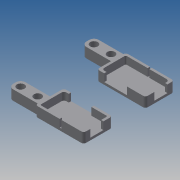
# Autodesk Inventor part: Limit Switch Mount Mount
Saved by Autodesk Inventor 2014 SP1 (Build 180222100, 222)
## iProperties
Created: 2014-02-14
Part Number: Limit Switch Mount Mount
Material: Generic
Document SubType Name: Modeling
Designer: Pradhan Alexander
Density: 1 g/cm^3
Appearance: Default
Author: Pradhan Alexander
Autodesk Inventor part; units mm, degrees
ref_plane "YZ Plane" through (0, 0, 0) normal (1, 0, 0) x (0, 1, 0)
ref_plane "XZ Plane" through (0, 0, 0) normal (0, 1, 0) x (-1, 0, 0)
ref_plane "XY Plane" through (0, 0, 0) normal (0, 0, 1) x (1, 0, 0)
sketch "Sketch1" plane through (0, 0, 0) normal (0, 1, 0) x (-1, 0, 0)
  line L0 (-4.3352, 9.4071) -> (21.4966, 9.4071)
  line L1 (23.2873, 7.6164) -> (23.2873, -4.8804)
  line L2 (20.7346, -6.5949) -> (-4.3352, -6.5949)
  line L3 (-5.9227, -5.0074) -> (-5.9227, 7.8196)
  line L4 (-5.9227, 10.9946) -> (23.2873, 10.9946)
  line L5 (24.8748, 9.4071) -> (24.8748, -6.5949)
  line L6 (23.2873, -8.1824) -> (-5.9227, -8.1824)
  line L7 (-7.5102, -6.5949) -> (-7.5102, 9.4071)
  arc A0 (-5.9227, -5.0074) -> (-4.3352, -6.5949) centre (-4.3352, -5.0074) ccw
  arc A1 (23.2873, 7.6164) -> (21.4966, 9.4071) centre (21.4966, 7.6164) ccw
  arc A2 (-7.5102, -6.5949) -> (-5.9227, -8.1824) centre (-5.9227, -6.5949) ccw
  arc A3 (-5.9227, 10.9946) -> (-7.5102, 9.4071) centre (-5.9227, 9.4071) ccw
  arc A4 (24.8748, 9.4071) -> (23.2873, 10.9946) centre (23.2873, 9.4071) ccw
  arc A5 (23.2873, -8.1824) -> (24.8748, -6.5949) centre (23.2873, -6.5949) ccw
  line L8 (-4.3352, 9.4071) -> (-5.129, 9.4071)
  line L9 (-5.9227, 8.6134) -> (-5.9227, 7.8196)
  line L10 (20.7346, -6.5949) -> (22.4935, -6.5949)
  line L11 (23.2873, -5.8011) -> (23.2873, -4.8804)
  arc A6 (22.4935, -6.5949) -> (23.2873, -5.8011) centre (22.4935, -5.8011) ccw
  arc A7 (-5.129, 9.4071) -> (-5.9227, 8.6134) centre (-5.129, 8.6134) ccw
  point P0 (-5.9227, 9.4071)
  point P1 (-5.9227, -6.5949)
  dimension "d0" = 16.002
  dimension "d2" = 1.5875
  dimension "d3" = 1.5875
  dimension "d4" = 1.5875
  dimension "d5" = 1.5875
  dimension "d31" = 0.7937
  dimension "d45" = 29.21
  constraints: 24 end point, 16 point on circle, 16 tangent, 10 point on line, 8 centre point, 4 parallel, 4 perpendicular, 2 equal radius, 2 horizontal, 1 collinear
  measures "d0" distance of point (-5.923, -6.595) point (-5.923, 9.407)
  measures "d2" distance between parallel lines of L3 L7
  measures "d3" distance between parallel lines of L5 L1
  measures "d4" distance between parallel lines of L6 L2
  measures "d5" distance between parallel lines of L0 L4
  measures "d31" radius of A6
  measures "d45" distance between parallel lines of L1 L3
extrude "Extrusion1" add sketch "Sketch1" along normal blind 6.35 contours L0 A1 L1 L11 A6 L10 L2 A0 L3 L9 A7 L8 | L4 A4 L5 A5 L6 A2 L7 A3
sketch "Sketch3" plane through (0, 6.35, 0) normal (0, 1, 0) x (1, 0, 0)
  line L0 (7.5102, -9.4071) -> (7.5102, 6.5949) projected
  arc A0 (7.5102, 6.5949) -> (5.9227, 8.1824) centre (5.9227, 6.5949) ccw projected
  line L1 (5.9227, 8.1824) -> (-23.2873, 8.1824) projected
  arc A1 (-23.2873, 8.1824) -> (-24.8748, 6.5949) centre (-23.2873, 6.5949) ccw projected
  line L2 (-24.8748, 6.5949) -> (-24.8748, -9.4071) projected
  arc A2 (-24.8748, -9.4071) -> (-23.2873, -10.9946) centre (-23.2873, -9.4071) ccw projected
  line L3 (-23.2873, -10.9946) -> (5.9227, -10.9946) projected
  arc A3 (5.9227, -10.9946) -> (7.5102, -9.4071) centre (5.9227, -9.4071) ccw projected
  line L4 (-4.3352, 6.5949) -> (4.132, 6.5949)
  line L5 (5.9227, 4.8042) -> (5.9227, -7.6926)
  line L6 (4.005, -9.4071) -> (-21.6998, -9.4071)
  line L7 (-23.2873, -7.8196) -> (-23.2873, 5.0074)
  line L8 (-23.2873, 8.1824) -> (5.9227, 8.1824)
  line L9 (7.5102, 6.5949) -> (7.5102, -9.4071)
  line L10 (5.9227, -10.9946) -> (-23.2873, -10.9946)
  line L11 (-24.8748, -9.4071) -> (-24.8748, 6.5949)
  arc A4 (-23.2873, -7.8196) -> (-21.6998, -9.4071) centre (-21.6998, -7.8196) ccw
  arc A5 (5.9227, 4.8042) -> (4.132, 6.5949) centre (4.132, 4.8042) ccw
  arc A6 (-24.8748, -9.4071) -> (-23.2873, -10.9946) centre (-23.2873, -9.4071) ccw
  arc A7 (-23.2873, 8.1824) -> (-24.8748, 6.5949) centre (-23.2873, 6.5949) ccw
  arc A8 (7.5102, 6.5949) -> (5.9227, 8.1824) centre (5.9227, 6.5949) ccw
  arc A9 (5.9227, -10.9946) -> (7.5102, -9.4071) centre (5.9227, -9.4071) ccw
  line L12 (-4.3352, 6.5949) -> (-22.4935, 6.5949)
  line L13 (-23.2873, 5.8011) -> (-23.2873, 5.0074)
  line L14 (4.005, -9.4071) -> (5.129, -9.4071)
  line L15 (5.9227, -8.6134) -> (5.9227, -7.6926)
  arc A10 (5.129, -9.4071) -> (5.9227, -8.6134) centre (5.129, -8.6134) ccw
  arc A11 (-22.4935, 6.5949) -> (-23.2873, 5.8011) centre (-22.4935, 5.8011) ccw
  point P0 (-23.2873, 6.5949)
  point P1 (5.9227, 6.5949)
  point P2 (-23.2873, -9.4071)
  dimension "d53" = 16.002
  dimension "d54" = 1.5875
  dimension "d55" = 1.5875
  dimension "d56" = 1.5875
  dimension "d57" = 1.5875
  dimension "d58" = 0.7937
  dimension "d59" = 29.21
  constraints: 24 end point, 16 point on circle, 16 tangent, 10 point on line, 8 centre point, 4 parallel, 4 perpendicular, 3 collinear, 2 equal radius, 2 horizontal
  measures "d53" distance of point (-23.287, -9.407) point (-23.287, 6.595)
  measures "d54" distance between parallel lines of L7 L11
  measures "d55" distance between parallel lines of L9 L5
  measures "d56" distance between parallel lines of L10 L6
  measures "d57" distance between parallel lines of L4 L8
  measures "d58" radius of A10
  measures "d59" distance between parallel lines of L5 L7
extrude "Extrusion8" cut sketch "Sketch3" against normal blind 4.7625 contours L4 A5 L5 L15 A10 L14 L6 A4 L7 L13 A11 L12
sketch "Sketch10" plane through (-23.2873, 0, 10.9946) normal (0, 0, 1) x (1, 0, 0)
  line L0 (29.21, 0) -> (29.21, 6.35) projected
  line L1 (0, 0) -> (0, 6.35) projected
  line L2 (0.7938, 6.35) -> (27.4193, 6.35) projected
  line L3 (0.7938, 1.5875) -> (27.4193, 1.5875) projected
  line L4 (3.175, 6.35) -> (18.415, 6.35)
  line L5 (18.415, 6.35) -> (18.415, 1.5875)
  line L6 (18.415, 1.5875) -> (3.175, 1.5875)
  line L7 (3.175, 1.5875) -> (3.175, 6.35)
  dimension "d62" = 10.795
  dimension "d63" = 3.175
  constraints: 8 end point, 2 parallel, 2 point on line, 1 horizontal, 1 perpendicular
  measures "d62" distance between parallel lines of L0 L5
  measures "d63" distance between parallel lines of L1 L7
extrude "Extrusion9" cut sketch "Sketch10" against normal blind 1.5875
sketch "Sketch11" plane through (7.5102, 0, 9.4071) normal (1, 0, 0) x (0, 0, -1)
  line L0 (0, 6.35) -> (16.002, 6.35) projected
  line L1 (0, 0) -> (0, 6.35) projected
  line L2 (1.5875, 1.5875) -> (15.2082, 1.5875) projected
  line L3 (4.318, 6.35) -> (13.208, 6.35)
  line L4 (13.208, 6.35) -> (13.208, 1.5875)
  line L5 (13.208, 1.5875) -> (4.318, 1.5875)
  line L6 (4.318, 1.5875) -> (4.318, 6.35)
  dimension "d66" = 4.318
  dimension "d67" = 8.89
  constraints: 8 end point, 2 parallel, 2 point on line, 1 horizontal, 1 perpendicular
  measures "d66" distance between parallel lines of L1 L6
  measures "d67" distance between parallel lines of L4 L6
extrude "Extrusion10" cut sketch "Sketch11" against normal blind 1.5875
sketch "Sketch12" plane through (5.9227, 0, -8.1824) normal (0, 0, -1) x (-1, 0, 0)
  line L0 (29.21, 0) -> (29.21, 6.35) projected
  line L1 (28.4162, 6.35) -> (1.7907, 6.35) projected
  line L2 (28.4162, 1.5875) -> (1.7907, 1.5875) projected
  line L3 (13.335, 6.35) -> (14.478, 6.35)
  line L4 (14.478, 6.35) -> (14.478, 1.5875)
  line L5 (14.478, 1.5875) -> (13.335, 1.5875)
  line L6 (13.335, 1.5875) -> (13.335, 6.35)
  dimension "d70" = 1.143
  dimension "d71" = 14.732
  constraints: 8 end point, 2 parallel, 2 point on line, 1 horizontal, 1 perpendicular
  measures "d70" distance between parallel lines of L4 L6
  measures "d71" distance between parallel lines of L4 L0
extrude "Extrusion11" cut sketch "Sketch12" against normal blind 1.5875
sketch "Sketch13" plane through (-24.8748, 0, -6.5949) normal (-1, 0, 0) x (0, 0, 1)
  line L0 (2.794, 1.5875) -> (11.684, 1.5875) projected
  line L1 (0, 0) -> (8.255, 0)
  line L2 (8.255, 0) -> (8.255, 1.5875)
  line L3 (8.255, 1.5875) -> (0, 1.5875)
  line L4 (0, 1.5875) -> (0, 0)
  dimension "d74" = 8.255
  dimension "d83" = 1.5875
  constraints: 8 end point, 2 parallel, 1 horizontal, 1 perpendicular, 1 point on line
  measures "d74" distance between parallel lines of L2 L4
  measures "d83" distance of L1.end L2.end
extrude "Extrusion12" add sketch "Sketch13" along normal blind 19.685
sketch "Sketch14" plane through (-24.8748, 1.5875, 1.6601) normal (0, 1, 0) x (1, 0, 0)
  line L0 (0, 8.255) -> (0, 0) projected
  line L1 (-19.685, 0) -> (-19.685, 8.255) projected
  circle A0 centre (-15.5575, 4.1275) radius 2.54
  circle A1 centre (-4.1275, 4.1275) radius 2.54
  point P0 (-19.685, 4.1275)
  dimension "d77" = 5.08
  dimension "d78" = 5.08
  dimension "d79" = 4.1275
  dimension "d80" = 4.1275
  constraints: 2 centre point, 2 horizontal alignment, 1 midpoint
  measures "d77" diameter of A0
  measures "d78" diameter of A1
  measures "d79" distance from line of L1 A0.centre
  measures "d80" distance from line of L0 A1.centre
extrude "Extrusion13" cut sketch "Sketch14" against normal blind 1.5875
fillet "Fillet2" radius 3.175 2 edges at (-44.5598, 0.7937, 1.6601) (-44.5598, 0.7937, -6.5949)
sketch "Sketch15" plane through (-24.8748, 1.5875, 1.6601) normal (0, 1, 0) x (1, 0, 0)
  circle A0 centre (-15.5575, 4.1275) radius 2.54 projected
  circle A1 centre (-4.1275, 4.1275) radius 2.54 projected
  arc A2 (-16.51, 8.255) -> (-19.685, 5.08) centre (-16.51, 5.08) ccw projected
  line L0 (-19.685, 3.175) -> (-19.685, 5.08) projected
  arc A3 (-19.685, 3.175) -> (-16.51, 0) centre (-16.51, 3.175) ccw projected
  line L1 (0, 0) -> (-16.51, 0) projected
  line L2 (0, 8.255) -> (0, 0) projected
  line L3 (0, 8.255) -> (-16.51, 8.255) projected
extrude "Extrusion14" add sketch "Sketch15" along normal blind 4.7625
sketch "Sketch16" plane through (7.5102, 0, 9.4071) normal (1, 0, 0) x (0, 0, -1)
  line L0 (4.318, 1.5875) -> (4.318, 6.35) projected
  line L1 (0, 6.35) -> (4.318, 6.35) projected
  line L2 (0, 0) -> (0, 6.35) projected
  line L3 (16.002, 0) -> (0, 0) projected
  line L4 (16.002, 0) -> (16.002, 6.35) projected
  line L5 (13.208, 6.35) -> (16.002, 6.35) projected
  line L6 (13.208, 6.35) -> (13.208, 1.5875) projected
  line L7 (13.208, 1.5875) -> (4.318, 1.5875) projected
  line L8 (0, 0) -> (-12.7, 0)
  line L9 (-1.5875, 0) -> (0, 0) projected
  dimension "d87" = 12.7
  constraints: 2 end point, 1 collinear
  measures "d87" distance of L2.start L8.end
ref_plane "Work Plane4" through (7.5102, 0, 22.1071) normal (0, 0, 1) x (1, 0, 0)
mirror "Mirror2" about plane through (7.5102, 0, 22.1071) normal (0, 0, 1) of "Extrusion1", "Extrusion8", "Extrusion9", "Extrusion10", "Extrusion11", "Extrusion12", "Extrusion13", "Fillet2", "Extrusion14"
sketch "Sketch17" plane through (0, 6.35, 0) normal (0, 1, 0) x (1, 0, 0)
  circle A0 centre (-40.4323, 2.4674) radius 2.54 projected
  circle A1 centre (-29.0023, 2.4674) radius 2.54 projected
  line L0 (-8.5553, 6.5949) -> (-8.5553, 8.1824) projected
  line L1 (-8.5553, 8.1824) -> (-23.2873, 8.1824) projected
  arc A2 (-23.2873, 8.1824) -> (-24.8748, 6.5949) centre (-23.2873, 6.5949) ccw projected
  line L2 (-24.8748, 6.5949) -> (-41.3848, 6.5949) projected
  arc A3 (-41.3848, 6.5949) -> (-44.5598, 3.4199) centre (-41.3848, 3.4199) ccw projected
  line L3 (-44.5598, 3.4199) -> (-44.5598, 1.5149) projected
  arc A4 (-44.5598, 1.5149) -> (-41.3848, -1.6601) centre (-41.3848, 1.5149) ccw projected
  line L4 (-41.3848, -1.6601) -> (-24.8748, -1.6601) projected
  line L5 (-24.8748, -1.6601) -> (-24.8748, -9.4071) projected
  arc A5 (-24.8748, -9.4071) -> (-23.2873, -10.9946) centre (-23.2873, -9.4071) ccw projected
  line L6 (-23.2873, -10.9946) -> (-20.1123, -10.9946) projected
  line L7 (-20.1123, -10.9946) -> (-20.1123, -9.4071) projected
  line L8 (-20.1123, -9.4071) -> (-21.6998, -9.4071) projected
  arc A6 (-23.2873, -7.8196) -> (-21.6998, -9.4071) centre (-21.6998, -7.8196) ccw projected
  line L9 (-23.2873, -7.8196) -> (-23.2873, 5.8011) projected
  arc A7 (-22.4935, 6.5949) -> (-23.2873, 5.8011) centre (-22.4935, 5.8011) ccw projected
  line L10 (-22.4935, 6.5949) -> (-8.5553, 6.5949) projected
  line L11 (-7.4123, 8.1824) -> (-7.4123, 6.5949) projected
  line L12 (-7.4123, 6.5949) -> (4.132, 6.5949) projected
  arc A8 (5.9227, 4.8042) -> (4.132, 6.5949) centre (4.132, 4.8042) ccw projected
  line L13 (5.9227, 4.8042) -> (5.9227, 3.8009) projected
  line L14 (5.9227, 3.8009) -> (7.5102, 3.8009) projected
  line L15 (7.5102, 3.8009) -> (7.5102, 6.5949) projected
  arc A9 (7.5102, 6.5949) -> (5.9227, 8.1824) centre (5.9227, 6.5949) ccw projected
  line L16 (5.9227, 8.1824) -> (-7.4123, 8.1824) projected
  line L17 (7.5102, -5.0891) -> (5.9227, -5.0891) projected
  line L18 (5.9227, -5.0891) -> (5.9227, -8.6134) projected
  arc A10 (5.129, -9.4071) -> (5.9227, -8.6134) centre (5.129, -8.6134) ccw projected
  line L19 (5.129, -9.4071) -> (-4.8723, -9.4071) projected
  line L20 (-4.8723, -9.4071) -> (-4.8723, -10.9946) projected
  line L21 (-4.8723, -10.9946) -> (5.9227, -10.9946) projected
  arc A11 (5.9227, -10.9946) -> (7.5102, -9.4071) centre (5.9227, -9.4071) ccw projected
  line L22 (7.5102, -9.4071) -> (7.5102, -5.0891) projected
  circle A12 centre (-40.4323, -46.6816) radius 2.54 projected
  circle A13 centre (-29.0023, -46.6816) radius 2.54 projected
  line L23 (-8.5553, -52.3966) -> (-8.5553, -50.8091) projected
  line L24 (-8.5553, -50.8091) -> (-22.4935, -50.8091) projected
  arc A14 (-23.2873, -50.0154) -> (-22.4935, -50.8091) centre (-22.4935, -50.0154) ccw projected
  line L25 (-23.2873, -50.0154) -> (-23.2873, -36.3946) projected
  arc A15 (-21.6998, -34.8071) -> (-23.2873, -36.3946) centre (-21.6998, -36.3946) ccw projected
  line L26 (-21.6998, -34.8071) -> (-20.1123, -34.8071) projected
  line L27 (-20.1123, -34.8071) -> (-20.1123, -33.2196) projected
  line L28 (-23.2873, -33.2196) -> (-20.1123, -33.2196) projected
  arc A16 (-23.2873, -33.2196) -> (-24.8748, -34.8071) centre (-23.2873, -34.8071) ccw projected
  line L29 (-24.8748, -42.5541) -> (-24.8748, -34.8071) projected
  line L30 (-41.3848, -42.5541) -> (-24.8748, -42.5541) projected
  arc A17 (-41.3848, -42.5541) -> (-44.5598, -45.7291) centre (-41.3848, -45.7291) ccw projected
  line L31 (-44.5598, -47.6341) -> (-44.5598, -45.7291) projected
  arc A18 (-44.5598, -47.6341) -> (-41.3848, -50.8091) centre (-41.3848, -47.6341) ccw projected
  line L32 (-24.8748, -50.8091) -> (-41.3848, -50.8091) projected
  arc A19 (-24.8748, -50.8091) -> (-23.2873, -52.3966) centre (-23.2873, -50.8091) ccw projected
  line L33 (-8.5553, -52.3966) -> (-23.2873, -52.3966) projected
  line L34 (5.9227, -39.1251) -> (7.5102, -39.1251) projected
  line L35 (7.5102, -34.8071) -> (7.5102, -39.1251) projected
  arc A20 (7.5102, -34.8071) -> (5.9227, -33.2196) centre (5.9227, -34.8071) ccw projected
  line L36 (-4.8723, -33.2196) -> (5.9227, -33.2196) projected
  line L37 (-4.8723, -33.2196) -> (-4.8723, -34.8071) projected
  line L38 (-4.8723, -34.8071) -> (5.129, -34.8071) projected
  arc A21 (5.9227, -35.6009) -> (5.129, -34.8071) centre (5.129, -35.6009) ccw projected
  line L39 (5.9227, -35.6009) -> (5.9227, -39.1251) projected
  line L40 (-7.4123, -50.8091) -> (-7.4123, -52.3966) projected
  line L41 (5.9227, -52.3966) -> (-7.4123, -52.3966) projected
  arc A22 (5.9227, -52.3966) -> (7.5102, -50.8091) centre (5.9227, -50.8091) ccw projected
  line L42 (7.5102, -48.0151) -> (7.5102, -50.8091) projected
  line L43 (7.5102, -48.0151) -> (5.9227, -48.0151) projected
  line L44 (5.9227, -48.0151) -> (5.9227, -49.0184) projected
  arc A23 (4.132, -50.8091) -> (5.9227, -49.0184) centre (4.132, -49.0184) ccw projected
  line L45 (4.132, -50.8091) -> (-7.4123, -50.8091) projected
extrude "Extrusion15" add sketch "Sketch17" along normal blind 0.3048
body "Solid1"
